Autodesk Fusion 360 part; units mm, degrees
(part 2 of 2)
  arc A410 through (-10.393, 21.7923, -1.2301) (-10.4251, 21.7969, -1.2301) (-10.4574, 21.7984, -1.2301)
  arc A411 through (-24.288, 21.2058, -1.2301) (-24.2358, 20.2463, -1.2301) (-24.1815, 19.2869, -1.2301)
  arc A412 through (-8.9436, 19.8011, -1.2301) (-8.8997, 19.8219, -1.2301) (-8.8672, 19.8581, -1.2301)
  arc A413 through (-23.6188, 17.8727, -1.2301) (-23.6343, 18.3175, -1.2301) (-23.6522, 18.7623, -1.2301)
  arc A414 through (-9.5131, 19.7961, -1.2301) (-9.3106, 19.7881, -1.2301) (-9.108, 19.7825, -1.2301)
  arc A415 through (-8.8381, 19.9649, -1.2301) (-8.8465, 20.0211, -1.2301) (-8.8708, 20.0725, -1.2301)
  arc A416 through (-10.2305, 21.4094, -1.2301) (-10.2433, 21.5149, -1.2301) (-10.2648, 21.619, -1.2301)
  arc A417 through (-8.8672, 19.8581, -1.2301) (-8.8455, 19.9096, -1.2301) (-8.8381, 19.9649, -1.2301)
  arc A418 through (-23.0477, 20.5417, -1.2301) (-22.9869, 20.5553, -1.2301) (-22.9246, 20.5568, -1.2301)
  arc A419 through (-23.9426, 17.1473, -1.2301) (-23.9119, 17.1378, -1.2301) (-23.8802, 17.1321, -1.2301)
  arc A420 through (-24.1815, 19.2869, -1.2301) (-24.1249, 18.3218, -1.2301) (-24.0665, 17.3569, -1.2301)
  arc A421 through (-20.1417, 17.4613, -1.2301) (-20.1217, 17.6929, -1.2301) (-20.123, 17.9253, -1.2301)
  arc A422 through (-29.5876, 20.7478, -1.2301) (-29.7687, 20.7693, -1.2301) (-29.9508, 20.7783, -1.2301)
  arc A423 through (-8.8708, 20.0725, -1.2301) (-8.9093, 20.1152, -1.2301) (-8.9583, 20.1453, -1.2301)
  arc A424 through (-22.2279, 17.2548, -1.2301) (-22.2157, 17.2128, -1.2301) (-22.1903, 17.1771, -1.2301)
  arc A425 through (-22.6634, 20.417, -1.2301) (-22.5849, 20.342, -1.2301) (-22.5222, 20.2535, -1.2301)
  arc A426 through (-22.4438, 20.0412, -1.2301) (-22.4151, 19.8563, -1.2301) (-22.3982, 19.6701, -1.2301)
  line L57 (-10.18, 20.3454, -1.2301) -> (-10.209, 21.0541, -1.2301)
  arc A427 through (-23.2603, 20.4621, -1.2301) (-23.1547, 20.5039, -1.2301) (-23.0477, 20.5417, -1.2301)
  arc A428 through (-23.6237, 17.4644, -1.2301) (-23.6167, 17.6685, -1.2301) (-23.6188, 17.8727, -1.2301)
  arc A429 through (-23.5247, 20.3582, -1.2301) (-23.4617, 20.3815, -1.2301) (-23.3991, 20.4057, -1.2301)
  arc A430 through (-23.987, 17.1766, -1.2301) (-23.9664, 17.1596, -1.2301) (-23.9426, 17.1473, -1.2301)
  arc A431 through (-8.9583, 20.1453, -1.2301) (-9.046, 20.1772, -1.2301) (-9.137, 20.1984, -1.2301)
  arc A432 through (-23.3991, 20.4057, -1.2301) (-23.3295, 20.4336, -1.2301) (-23.2603, 20.4621, -1.2301)
  arc A433 through (-24.0665, 17.3569, -1.2301) (-24.0429, 17.2597, -1.2301) (-23.987, 17.1766, -1.2301)
  arc A434 through (-10.58, 21.7765, -1.2301) (-10.6003, 21.7661, -1.2301) (-10.618, 21.7517, -1.2301)
  arc A435 through (-10.1824, 19.8082, -1.2301) (-10.0878, 19.8088, -1.2301) (-9.9932, 19.809, -1.2301)
  arc A436 through (-21.5279, 20.4378, -1.2301) (-21.3194, 20.4978, -1.2301) (-21.1031, 20.5148, -1.2301)
  arc A437 through (-24.232, 21.4248, -1.2301) (-24.2767, 21.3196, -1.2301) (-24.288, 21.2058, -1.2301)
  arc A438 through (-22.5222, 20.2535, -1.2301) (-22.4741, 20.1506, -1.2301) (-22.4438, 20.0412, -1.2301)
  arc A439 through (-23.6307, 20.3208, -1.2301) (-23.5776, 20.3392, -1.2301) (-23.5247, 20.3582, -1.2301)
  arc A440 through (-22.8153, 20.5219, -1.2301) (-22.7378, 20.4718, -1.2301) (-22.6634, 20.417, -1.2301)
  line L58 (-9.509, 20.2552, -1.2301) -> (-10.18, 20.3454, -1.2301)
  arc A441 through (-29.9508, 20.7783, -1.2301) (-30.1091, 20.7741, -1.2301) (-30.2665, 20.7566, -1.2301)
  arc A442 through (-21.8313, 20.8664, -1.2301) (-21.9495, 20.8378, -1.2301) (-22.07, 20.8212, -1.2301)
  arc A443 through (-20.5452, 17.5083, -1.2301) (-20.5219, 17.4117, -1.2301) (-20.4913, 17.3172, -1.2301)
  arc A444 through (-20.3931, 20.5982, -1.2301) (-20.4399, 20.6955, -1.2301) (-20.5052, 20.7815, -1.2301)
  arc A445 through (-23.744, 20.8149, -1.2301) (-23.7527, 20.818, -1.2301) (-23.7576, 20.8258, -1.2301)
  arc A446 through (-20.3188, 20.319, -1.2301) (-20.35, 20.4602, -1.2301) (-20.3931, 20.5982, -1.2301)
  arc A447 through (-21.2466, 21.0547, -1.2301) (-21.4005, 21.0192, -1.2301) (-21.5495, 20.9666, -1.2301)
  arc A448 through (-20.8881, 10.6636, -1.2301) (-20.8934, 10.6501, -1.2301) (-20.9065, 10.6439, -1.2301)
  arc A449 through (-27.9096, 11.2292, -1.2301) (-27.9142, 11.2191, -1.2301) (-27.9245, 11.2149, -1.2301)
  line L59 (-29.0881, 10.6149, -1.2301) -> (-29.9881, 10.6149, -1.2301)
  arc A450 through (-28.743, 10.6184, -1.2301) (-28.9156, 10.6158, -1.2301) (-29.0881, 10.6149, -1.2301)
  arc A451 through (-23.1426, 13.9894, -1.2301) (-23.1567, 13.9402, -1.2301) (-23.1621, 13.8893, -1.2301)
  arc A452 through (-27.9245, 11.2149, -1.2301) (-27.9375, 11.2179, -1.2301) (-27.948, 11.2262, -1.2301)
  arc A453 through (-28.1881, 10.6636, -1.2301) (-28.1934, 10.6501, -1.2301) (-28.2065, 10.6439, -1.2301)
  line L60 (-29.799, 13.6149, -1.2301) -> (-28.8436, 13.6149, -1.2301)
  arc A454 through (-21.1525, 10.6292, -1.2301) (-21.2977, 10.6226, -1.2301) (-21.443, 10.6184, -1.2301)
  line L61 (-21.7881, 10.6149, -1.2301) -> (-22.6881, 10.6149, -1.2301)
  line L62 (-20.1381, 14.0649, -1.2301) -> (-21.6152, 14.0926, -1.2301)
  arc A455 through (-20.9065, 10.6439, -1.2301) (-21.0295, 10.6362, -1.2301) (-21.1525, 10.6292, -1.2301)
  arc A456 through (-28.7431, 11.4263, -1.2301) (-28.5972, 11.2334, -1.2301) (-28.4525, 11.0398, -1.2301)
  line L63 (-23.1381, 10.1649, -1.2301) -> (-21.6381, 10.1649, -1.2301)
  arc A457 through (-23.1723, 12.7289, -1.2301) (-23.1698, 12.3703, -1.2301) (-23.1655, 12.0117, -1.2301)
  arc A458 through (-22.7937, 14.0871, -1.2301) (-22.9279, 14.0747, -1.2301) (-23.0614, 14.0557, -1.2301)
  line L64 (-21.5799, 12.4149, -1.2301) -> (-22.499, 13.6149, -1.2301)
  line L65 (-28.8799, 12.4149, -1.2301) -> (-29.799, 13.6149, -1.2301)
  line L66 (-20.5881, 13.6149, -1.2301) -> (-20.5881, 12.4149, -1.2301)
  arc A459 through (-27.948, 11.2262, -1.2301) (-28.0841, 11.3968, -1.2301) (-28.2201, 11.5674, -1.2301)
  line L67 (-22.6881, 10.6149, -1.2301) -> (-22.6881, 11.8272, -1.2301)
  arc A460 through (-28.1995, 10.6981, -1.2301) (-28.191, 10.6817, -1.2301) (-28.1881, 10.6636, -1.2301)
  arc A461 through (-20.648, 11.2262, -1.2301) (-20.7841, 11.3968, -1.2301) (-20.9201, 11.5674, -1.2301)
  line L68 (-21.6381, 10.1649, -1.2301) -> (-20.1381, 10.1649, -1.2301)
  arc A462 through (-21.6152, 14.0926, -1.2301) (-21.9888, 14.0982, -1.2301) (-22.3625, 14.1009, -1.2301)
  line L69 (-29.9881, 10.6149, -1.2301) -> (-29.9881, 11.8272, -1.2301)
  arc A463 through (-21.2249, 11.9549, -1.2301) (-21.4028, 12.1846, -1.2301) (-21.5799, 12.4149, -1.2301)
  arc A464 through (-28.2201, 11.5674, -1.2301) (-28.3731, 11.7607, -1.2301) (-28.5249, 11.9549, -1.2301)
  line L70 (-22.499, 13.6149, -1.2301) -> (-21.5436, 13.6149, -1.2301)
  line L71 (-29.9881, 13.0395, -1.2301) -> (-29.0881, 11.8758, -1.2301)
  line L72 (-23.1655, 12.0117, -1.2301) -> (-23.1381, 10.1649, -1.2301)
  arc A465 through (-21.4431, 11.4263, -1.2301) (-21.2972, 11.2334, -1.2301) (-21.1525, 11.0398, -1.2301)
  arc A466 through (-27.8881, 12.4149, -1.2301) (-27.8888, 12.1849, -1.2301) (-27.8907, 11.9548, -1.2301)
  arc A467 through (-21.1525, 11.0398, -1.2301) (-21.0259, 10.869, -1.2301) (-20.8995, 10.6981, -1.2301)
  arc A468 through (-18.1458, 13.994, -1.2301) (-18.1575, 13.8838, -1.2301) (-18.1675, 13.7735, -1.2301)
  arc A469 through (-18.1675, 13.7735, -1.2301) (-18.1769, 13.6401, -1.2301) (-18.183, 13.5064, -1.2301)
  arc A470 through (-18.118, 14.0517, -1.2301) (-18.1368, 14.0252, -1.2301) (-18.1458, 13.994, -1.2301)
  line L73 (-29.9881, 11.8272, -1.2301) -> (-29.9881, 13.0395, -1.2301)
  line L74 (-28.8436, 13.6149, -1.2301) -> (-27.8881, 13.6149, -1.2301)
  line L75 (-22.6881, 13.0395, -1.2301) -> (-21.7881, 11.8758, -1.2301)
  arc A471 through (-27.8907, 11.9548, -1.2301) (-27.8939, 11.7611, -1.2301) (-27.8988, 11.5674, -1.2301)
  arc A472 through (-20.5988, 11.5674, -1.2301) (-20.6041, 11.3983, -1.2301) (-20.6096, 11.2292, -1.2301)
  arc A473 through (-30.3614, 14.0557, -1.2301) (-30.4108, 14.0334, -1.2301) (-30.4426, 13.9894, -1.2301)
  arc A474 through (-28.4525, 11.0398, -1.2301) (-28.3259, 10.869, -1.2301) (-28.1995, 10.6981, -1.2301)
  arc A475 through (-27.8988, 11.5674, -1.2301) (-27.9041, 11.3983, -1.2301) (-27.9096, 11.2292, -1.2301)
  arc A476 through (-28.2065, 10.6439, -1.2301) (-28.3295, 10.6362, -1.2301) (-28.4525, 10.6292, -1.2301)
  arc A477 through (-21.7881, 11.8758, -1.2301) (-21.6152, 11.6514, -1.2301) (-21.4431, 11.4263, -1.2301)
  arc A478 through (-20.9201, 11.5674, -1.2301) (-21.0731, 11.7607, -1.2301) (-21.2249, 11.9549, -1.2301)
  arc A479 through (-20.8995, 10.6981, -1.2301) (-20.891, 10.6817, -1.2301) (-20.8881, 10.6636, -1.2301)
  arc A480 through (-29.0881, 11.8758, -1.2301) (-28.9152, 11.6514, -1.2301) (-28.7431, 11.4263, -1.2301)
  arc A481 through (-20.5907, 11.9548, -1.2301) (-20.5939, 11.7611, -1.2301) (-20.5988, 11.5674, -1.2301)
  arc A482 through (-28.4525, 10.6292, -1.2301) (-28.5977, 10.6226, -1.2301) (-28.743, 10.6184, -1.2301)
  arc A483 through (-20.5881, 12.4149, -1.2301) (-20.5888, 12.1849, -1.2301) (-20.5907, 11.9548, -1.2301)
  arc A484 through (-20.6245, 11.2149, -1.2301) (-20.6375, 11.2179, -1.2301) (-20.648, 11.2262, -1.2301)
  arc A485 through (-23.17, 13.3545, -1.2301) (-23.1724, 13.0417, -1.2301) (-23.1723, 12.7289, -1.2301)
  arc A486 through (-21.443, 10.6184, -1.2301) (-21.6156, 10.6158, -1.2301) (-21.7881, 10.6149, -1.2301)
  line L76 (-20.1381, 10.1649, -1.2301) -> (-20.1381, 12.1149, -1.2301)
  line L77 (-22.6881, 11.8272, -1.2301) -> (-22.6881, 13.0395, -1.2301)
  arc A487 through (-22.3625, 14.1009, -1.2301) (-22.5782, 14.0978, -1.2301) (-22.7937, 14.0871, -1.2301)
  arc A488 through (-23.0614, 14.0557, -1.2301) (-23.1108, 14.0334, -1.2301) (-23.1426, 13.9894, -1.2301)
  arc A489 through (-28.5249, 11.9549, -1.2301) (-28.7028, 12.1846, -1.2301) (-28.8799, 12.4149, -1.2301)
  arc A490 through (-20.6096, 11.2292, -1.2301) (-20.6142, 11.2191, -1.2301) (-20.6245, 11.2149, -1.2301)
  arc A491 through (-23.1621, 13.8893, -1.2301) (-23.1665, 13.6219, -1.2301) (-23.17, 13.3545, -1.2301)
  line L78 (-27.8881, 13.6149, -1.2301) -> (-27.8881, 12.4149, -1.2301)
  arc A492 through (-30.0937, 14.0871, -1.2301) (-30.2279, 14.0747, -1.2301) (-30.3614, 14.0557, -1.2301)
  line L79 (-20.1381, 12.1149, -1.2301) -> (-20.1381, 14.0649, -1.2301)
  line L80 (-21.5436, 13.6149, -1.2301) -> (-20.5881, 13.6149, -1.2301)
  arc A493 through (-18.0469, 10.2033, -1.2301) (-17.9958, 10.1748, -1.2301) (-17.9381, 10.1649, -1.2301)
  arc A494 through (-16.7055, 12.3715, -1.2301) (-16.8822, 12.3846, -1.2301) (-17.0592, 12.3946, -1.2301)
  line L81 (-18.1958, 11.9056, -1.2301) -> (-18.1669, 11.0353, -1.2301)
  line L82 (-18.8169, 11.9353, -1.2301) -> (-18.1958, 11.9056, -1.2301)
  line L83 (-17.6805, 11.9056, -1.2301) -> (-17.0593, 11.9353, -1.2301)
  line L84 (-18.1881, 13.203, -1.2301) -> (-18.1881, 12.4245, -1.2301)
  arc A495 through (-18.183, 13.5064, -1.2301) (-18.1868, 13.3548, -1.2301) (-18.1881, 13.203, -1.2301)
  arc A496 through (-19.3313, 12.3358, -1.2301) (-19.3756, 12.3102, -1.2301) (-19.4089, 12.2713, -1.2301)
  arc A497 through (-16.5445, 11.9941, -1.2301) (-16.5003, 12.0197, -1.2301) (-16.4672, 12.0586, -1.2301)
  arc A498 through (-19.1707, 11.9584, -1.2301) (-18.9939, 11.9453, -1.2301) (-18.8169, 11.9353, -1.2301)
  arc A499 through (-19.4091, 12.0586, -1.2301) (-19.376, 12.0197, -1.2301) (-19.3318, 11.9941, -1.2301)
  arc A500 through (-10.3041, 13.1503, -1.2301) (-10.1609, 13.1636, -1.2301) (-10.0192, 13.1876, -1.2301)
  arc A501 through (-16.5445, 12.3358, -1.2301) (-16.6237, 12.3591, -1.2301) (-16.7055, 12.3715, -1.2301)
  arc A502 through (-17.0593, 11.9353, -1.2301) (-16.8823, 11.9453, -1.2301) (-16.7055, 11.9584, -1.2301)
  arc A503 through (-15.1512, 10.2264, -1.2301) (-15.1025, 10.1813, -1.2301) (-15.0381, 10.1649, -1.2301)
  arc A504 through (-16.7055, 11.9584, -1.2301) (-16.6238, 11.9707, -1.2301) (-16.5445, 11.9941, -1.2301)
  arc A505 through (-18.023, 14.0926, -1.2301) (-18.0519, 14.0859, -1.2301) (-18.08, 14.0765, -1.2301)
  arc A506 through (-10.4908, 10.2591, -1.2301) (-10.2893, 10.2689, -1.2301) (-10.0887, 10.2893, -1.2301)
  line L85 (-17.7093, 11.0353, -1.2301) -> (-17.6805, 11.9056, -1.2301)
  arc A507 through (-17.7317, 10.5158, -1.2301) (-17.7192, 10.7755, -1.2301) (-17.7093, 11.0353, -1.2301)
  arc A508 through (-16.4672, 12.0586, -1.2301) (-16.4455, 12.1098, -1.2301) (-16.4381, 12.1649, -1.2301)
  arc A509 through (-12.7902, 11.1668, -1.2301) (-12.7379, 11.3526, -1.2301) (-12.6848, 11.5381, -1.2301)
  arc A510 through (-17.7305, 13.6633, -1.2301) (-17.7428, 13.7827, -1.2301) (-17.7639, 13.901, -1.2301)
  arc A511 through (-18.1111, 10.3023, -1.2301) (-18.0869, 10.2476, -1.2301) (-18.0469, 10.2033, -1.2301)
  arc A512 through (-10.407, 10.6709, -1.2301) (-10.885, 10.6828, -1.2301) (-11.3631, 10.6925, -1.2301)
  arc A513 through (-19.4381, 12.1649, -1.2301) (-19.4307, 12.1098, -1.2301) (-19.4091, 12.0586, -1.2301)
  arc A514 through (-12.8596, 10.7627, -1.2301) (-12.8791, 10.7722, -1.2301) (-12.8867, 10.7925, -1.2301)
  arc A515 through (-19.1694, 12.3715, -1.2301) (-19.2516, 12.3592, -1.2301) (-19.3313, 12.3358, -1.2301)
  arc A516 through (-15.0134, 13.5959, -1.2301) (-15.0488, 13.6, -1.2301) (-15.0843, 13.5986, -1.2301)
  arc A517 through (-16.4672, 12.2712, -1.2301) (-16.5003, 12.3102, -1.2301) (-16.5445, 12.3358, -1.2301)
  line L86 (-18.1881, 12.4245, -1.2301) -> (-18.8131, 12.3947, -1.2301)
  arc A518 through (-17.9381, 10.1649, -1.2301) (-17.8805, 10.1748, -1.2301) (-17.8294, 10.2033, -1.2301)
  arc A519 through (-17.7651, 10.3023, -1.2301) (-17.743, 10.4082, -1.2301) (-17.7317, 10.5158, -1.2301)
  arc A520 through (-18.8131, 12.3947, -1.2301) (-18.9914, 12.3847, -1.2301) (-19.1694, 12.3715, -1.2301)
  arc A521 through (-18.1669, 11.0353, -1.2301) (-18.157, 10.7755, -1.2301) (-18.1445, 10.5158, -1.2301)
  arc A522 through (-18.1445, 10.5158, -1.2301) (-18.1332, 10.4082, -1.2301) (-18.1111, 10.3023, -1.2301)
  arc A523 through (-9.8894, 13.4761, -1.2301) (-9.9521, 13.5166, -1.2301) (-10.0231, 13.5395, -1.2301)
  arc A524 through (-15.0381, 10.1649, -1.2301) (-14.9733, 10.182, -1.2301) (-14.9253, 10.2288, -1.2301)
  arc A525 through (-10.0231, 13.5395, -1.2301) (-10.169, 13.5606, -1.2301) (-10.3161, 13.571, -1.2301)
  arc A526 through (-13.0848, 11.9529, -1.2301) (-13.2769, 11.3044, -1.2301) (-13.4636, 10.6545, -1.2301)
  arc A527 through (-15.2726, 12.3824, -1.2301) (-15.2702, 12.0716, -1.2301) (-15.2658, 11.7609, -1.2301)
  arc A528 through (-19.3318, 11.9941, -1.2301) (-19.2525, 11.9707, -1.2301) (-19.1707, 11.9584, -1.2301)
  arc A529 through (-12.5967, 10.2277, -1.2301) (-12.106, 10.2314, -1.2301) (-11.6154, 10.2376, -1.2301)
  arc A530 through (-16.4381, 12.1649, -1.2301) (-16.4455, 12.22, -1.2301) (-16.4672, 12.2712, -1.2301)
  arc A531 through (-17.893, 14.0923, -1.2301) (-17.9251, 14.0969, -1.2301) (-17.9574, 14.0984, -1.2301)
  arc A532 through (-19.4089, 12.2713, -1.2301) (-19.4307, 12.2201, -1.2301) (-19.4381, 12.1649, -1.2301)
  arc A533 through (-9.8882, 13.2535, -1.2301) (-9.8512, 13.3039, -1.2301) (-9.8381, 13.3649, -1.2301)
  arc A534 through (-12.879, 10.8461, -1.2301) (-12.8347, 11.0065, -1.2301) (-12.7902, 11.1668, -1.2301)
  arc A535 through (-17.8294, 10.2033, -1.2301) (-17.7893, 10.2476, -1.2301) (-17.7651, 10.3023, -1.2301)
  line L87 (-12.2347, 13.0649, -1.2301) -> (-11.0364, 13.1149, -1.2301)
  arc A536 through (-13.0794, 10.2426, -1.2301) (-12.8382, 10.2308, -1.2301) (-12.5967, 10.2277, -1.2301)
  arc A537 through (-14.8662, 13.2955, -1.2301) (-14.8843, 13.4057, -1.2301) (-14.9158, 13.5127, -1.2301)
  arc A538 through (-15.1526, 13.5797, -1.2301) (-15.1817, 13.5636, -1.2301) (-15.2078, 13.5428, -1.2301)
  arc A539 through (-12.4397, 10.7333, -1.2301) (-12.6497, 10.7475, -1.2301) (-12.8596, 10.7627, -1.2301)
  arc A540 through (-12.5086, 13.4927, -1.2301) (-12.6164, 13.3803, -1.2301) (-12.6856, 13.2408, -1.2301)
  arc A541 through (-11.0364, 13.1149, -1.2301) (-10.6702, 13.1314, -1.2301) (-10.3041, 13.1503, -1.2301)
  arc A542 through (-17.9574, 14.0984, -1.2301) (-17.9903, 14.0969, -1.2301) (-18.023, 14.0926, -1.2301)
  arc A543 through (-9.8381, 10.4649, -1.2301) (-9.8539, 10.5287, -1.2301) (-9.8976, 10.5776, -1.2301)
  arc A544 through (-15.2658, 11.7609, -1.2301) (-15.256, 11.2591, -1.2301) (-15.2441, 10.7574, -1.2301)
  arc A545 through (-9.8381, 13.3649, -1.2301) (-9.8516, 13.4261, -1.2301) (-9.8894, 13.4761, -1.2301)
  arc A546 through (-13.4636, 10.6545, -1.2301) (-13.4808, 10.5065, -1.2301) (-13.4503, 10.3606, -1.2301)
  arc A547 through (-9.9044, 10.3508, -1.2301) (-9.8559, 10.3989, -1.2301) (-9.8381, 10.4649, -1.2301)
  arc A548 through (-14.8381, 11.8636, -1.2301) (-14.8393, 12.3675, -1.2301) (-14.8428, 12.8714, -1.2301)
  arc A549 through (-11.6154, 10.2376, -1.2301) (-11.0531, 10.2473, -1.2301) (-10.4908, 10.2591, -1.2301)
  arc A550 through (-10.0887, 10.2893, -1.2301) (-9.9935, 10.311, -1.2301) (-9.9044, 10.3508, -1.2301)
  line L88 (-17.0592, 12.3946, -1.2301) -> (-17.6802, 12.4243, -1.2301)
  arc A551 through (-15.0843, 13.5986, -1.2301) (-15.1192, 13.5918, -1.2301) (-15.1526, 13.5797, -1.2301)
  arc A552 through (-10.0192, 13.1876, -1.2301) (-9.9493, 13.212, -1.2301) (-9.8882, 13.2535, -1.2301)
  arc A553 through (-15.2699, 12.9281, -1.2301) (-15.2725, 12.6553, -1.2301) (-15.2726, 12.3824, -1.2301)
  arc A554 through (-18.08, 14.0765, -1.2301) (-18.1003, 14.0661, -1.2301) (-18.118, 14.0517, -1.2301)
  arc A555 through (-15.2411, 13.4933, -1.2301) (-15.2555, 13.4431, -1.2301) (-15.2612, 13.3913, -1.2301)
  arc A556 through (-14.8428, 12.8714, -1.2301) (-14.8497, 13.0838, -1.2301) (-14.8662, 13.2955, -1.2301)
  arc A557 through (-11.3631, 10.6925, -1.2301) (-11.6555, 10.6991, -1.2301) (-11.9478, 10.7083, -1.2301)
  arc A558 through (-15.2078, 13.5428, -1.2301) (-15.2272, 13.5199, -1.2301) (-15.2411, 13.4933, -1.2301)
  arc A559 through (-14.9253, 10.2288, -1.2301) (-14.8865, 10.3124, -1.2301) (-14.8661, 10.4023, -1.2301)
  line L89 (-17.6802, 12.4243, -1.2301) -> (-17.7092, 13.2435, -1.2301)
  arc A560 through (-10.3161, 13.571, -1.2301) (-10.7031, 13.583, -1.2301) (-11.0902, 13.5927, -1.2301)
  arc A561 through (-12.6856, 13.2408, -1.2301) (-12.8879, 12.5977, -1.2301) (-13.0848, 11.9529, -1.2301)
  arc A562 through (-13.3545, 10.2796, -1.2301) (-13.2176, 10.2565, -1.2301) (-13.0794, 10.2426, -1.2301)
  arc A563 through (-15.2612, 13.3913, -1.2301) (-15.2661, 13.1597, -1.2301) (-15.2699, 12.9281, -1.2301)
  arc A564 through (-9.8976, 10.5776, -1.2301) (-9.9739, 10.6179, -1.2301) (-10.0572, 10.6402, -1.2301)
  arc A565 through (-12.8867, 10.7925, -1.2301) (-12.8845, 10.8195, -1.2301) (-12.879, 10.8461, -1.2301)
  arc A566 through (-15.2135, 10.3929, -1.2301) (-15.1914, 10.3063, -1.2301) (-15.1512, 10.2264, -1.2301)
  arc A567 through (-17.8149, 14.036, -1.2301) (-17.8477, 14.0728, -1.2301) (-17.893, 14.0923, -1.2301)
  arc A568 through (-15.2441, 10.7574, -1.2301) (-15.2341, 10.5747, -1.2301) (-15.2135, 10.3929, -1.2301)
  arc A569 through (-10.0572, 10.6402, -1.2301) (-10.2316, 10.6608, -1.2301) (-10.407, 10.6709, -1.2301)
  arc A570 through (-14.8661, 10.4023, -1.2301) (-14.8489, 10.5928, -1.2301) (-14.8422, 10.7841, -1.2301)
  arc A571 through (-13.4503, 10.3606, -1.2301) (-13.4128, 10.3078, -1.2301) (-13.3545, 10.2796, -1.2301)
  line L90 (-12.56, 11.9649, -1.2301) -> (-12.2347, 13.0649, -1.2301)
  arc A572 through (-11.9478, 10.7083, -1.2301) (-12.1938, 10.719, -1.2301) (-12.4397, 10.7333, -1.2301)
  arc A573 through (-17.7092, 13.2435, -1.2301) (-17.7182, 13.4535, -1.2301) (-17.7305, 13.6633, -1.2301)
  arc A574 through (-14.8422, 10.7841, -1.2301) (-14.8391, 11.3238, -1.2301) (-14.8381, 11.8636, -1.2301)
  arc A575 through (-12.6848, 11.5381, -1.2301) (-12.6227, 11.7516, -1.2301) (-12.56, 11.9649, -1.2301)
  arc A576 through (-14.9158, 13.5127, -1.2301) (-14.9537, 13.5672, -1.2301) (-15.0134, 13.5959, -1.2301)
  arc A577 through (-17.7639, 13.901, -1.2301) (-17.7844, 13.9703, -1.2301) (-17.8149, 14.036, -1.2301)
  arc A578 through (-12.3707, 13.5523, -1.2301) (-12.4434, 13.5311, -1.2301) (-12.5086, 13.4927, -1.2301)
  arc A579 through (-5.303, 17.8735, -1.2301) (-5.3191, 18.4384, -1.2301) (-5.3405, 19.0032, -1.2301)
  arc A580 through (-5.439, 17.1788, -1.2301) (-5.3695, 17.2704, -1.2301) (-5.3339, 17.3797, -1.2301)
  arc A581 through (-7.9514, 16.9186, -1.2301) (-7.8874, 16.9218, -1.2301) (-7.8258, 16.9395, -1.2301)
  arc A582 through (-6.9071, 20.8063, -1.2301) (-6.7489, 20.8111, -1.2301) (-6.5938, 20.7795, -1.2301)
  arc A583 through (-12.0919, 13.5847, -1.2301) (-12.2317, 13.5716, -1.2301) (-12.3707, 13.5523, -1.2301)
  arc A584 through (-5.7471, 17.5199, -1.2301) (-5.7247, 17.3753, -1.2301) (-5.6952, 17.232, -1.2301)
  line L91 (-5.9074, 20.4105, -1.2301) -> (-5.8346, 18.8045, -1.2301)
  line L92 (-5.3405, 19.0032, -1.2301) -> (-5.4135, 20.7108, -1.2301)
  arc A585 through (-7.5304, 20.4229, -1.2301) (-7.3761, 20.5652, -1.2301) (-7.2079, 20.6906, -1.2301)
  line L93 (-5.4135, 20.7108, -1.2301) -> (-5.8722, 20.9796, -1.2301)
  arc A586 through (-7.7388, 17.0138, -1.2301) (-7.7224, 17.0517, -1.2301) (-7.7174, 17.0928, -1.2301)
  arc A587 through (-5.8722, 20.9796, -1.2301) (-5.9752, 21.0359, -1.2301) (-6.0815, 21.0858, -1.2301)
  arc A588 through (-5.8346, 18.8045, -1.2301) (-5.8145, 18.3956, -1.2301) (-5.7915, 17.9868, -1.2301)
  arc A589 through (-5.6182, 17.1435, -1.2301) (-5.5235, 17.1353, -1.2301) (-5.439, 17.1788, -1.2301)
  arc A590 through (-11.6862, 13.5991, -1.2301) (-11.8892, 13.5954, -1.2301) (-12.0919, 13.5847, -1.2301)
  arc A591 through (-8.4899, 21.1855, -1.2301) (-8.3522, 19.2872, -1.2301) (-8.2134, 17.389, -1.2301)
  arc A592 through (-7.2079, 20.6906, -1.2301) (-7.0639, 20.7652, -1.2301) (-6.9071, 20.8063, -1.2301)
  line L94 (-6.2345, 20.6127, -1.2301) -> (-5.9074, 20.4105, -1.2301)
  arc A593 through (-5.6952, 17.232, -1.2301) (-5.6678, 17.1781, -1.2301) (-5.6182, 17.1435, -1.2301)
  arc A594 through (-5.3339, 17.3797, -1.2301) (-5.3078, 17.6259, -1.2301) (-5.303, 17.8735, -1.2301)
  arc A595 through (-8.7308, 25.2268, -1.2301) (-8.7625, 25.1512, -1.2301) (-8.7695, 25.0694, -1.2301)
  arc A596 through (-11.0902, 13.5927, -1.2301) (-11.3882, 13.5976, -1.2301) (-11.6862, 13.5991, -1.2301)
  line L95 (-7.9132, 20.0308, -1.2301) -> (-7.5304, 20.4229, -1.2301)
  arc A597 through (-8.7695, 25.0694, -1.2301) (-8.63, 23.1274, -1.2301) (-8.4899, 21.1855, -1.2301)
  arc A598 through (-7.7547, 18.0055, -1.2301) (-7.7738, 18.2887, -1.2301) (-7.7954, 18.5718, -1.2301)
  arc A599 through (-33.8381, 22.9018, -1.2301) (-34.111, 22.8838, -1.2301) (-34.3838, 22.8645, -1.2301)
  arc A600 through (-27.0705, 23.1748, -1.2301) (-26.9835, 22.0437, -1.2301) (-26.8957, 20.9126, -1.2301)
  arc A601 through (-26.8957, 20.9126, -1.2301) (-26.8143, 19.895, -1.2301) (-26.7287, 18.8776, -1.2301)
  arc A602 through (-35.4029, 20.2744, -1.2301) (-35.3569, 19.4444, -1.2301) (-35.3035, 18.6149, -1.2301)
  arc A603 through (-35.4542, 22.6398, -1.2301) (-35.4522, 22.1115, -1.2301) (-35.4462, 21.5832, -1.2301)
  arc A604 through (-25.7292, 17.7001, -1.2301) (-25.8567, 17.7153, -1.2301) (-25.9629, 17.7874, -1.2301)
  arc A605 through (-7.7302, 17.5123, -1.2301) (-7.7408, 17.7589, -1.2301) (-7.7547, 18.0055, -1.2301)
  arc A606 through (-25.082, 17.7409, -1.2301) (-25.1883, 17.7492, -1.2301) (-25.2949, 17.7457, -1.2301)
  arc A607 through (-8.1393, 17.0399, -1.2301) (-8.112, 16.9918, -1.2301) (-8.0702, 16.9557, -1.2301)
  arc A608 through (-35.1482, 17.707, -1.2301) (-35.0971, 17.6758, -1.2301) (-35.0381, 17.6649, -1.2301)
  arc A609 through (-7.8258, 16.9395, -1.2301) (-7.7765, 16.9699, -1.2301) (-7.7388, 17.0138, -1.2301)
  arc A610 through (-5.7915, 17.9868, -1.2301) (-5.7734, 17.7529, -1.2301) (-5.7471, 17.5199, -1.2301)
  arc A611 through (-6.3319, 21.1825, -1.2301) (-6.4568, 21.2221, -1.2301) (-6.5831, 21.2566, -1.2301)
  line L96 (-7.7954, 18.5718, -1.2301) -> (-7.9132, 20.0308, -1.2301)
  arc A612 through (-35.3662, 22.7661, -1.2301) (-35.43, 22.7168, -1.2301) (-35.4542, 22.6398, -1.2301)
  arc A613 through (-8.5717, 25.2989, -1.2301) (-8.6056, 25.2952, -1.2301) (-8.6388, 25.2875, -1.2301)
  arc A614 through (-8.0702, 16.9557, -1.2301) (-8.013, 16.93, -1.2301) (-7.9514, 16.9186, -1.2301)
  line L97 (-7.9613, 20.7178, -1.2301) -> (-8.0894, 22.4914, -1.2301)
  arc A615 through (-24.9086, 17.5902, -1.2301) (-24.9298, 17.6455, -1.2301) (-24.9681, 17.6906, -1.2301)
  arc A616 through (-35.3035, 18.6149, -1.2301) (-35.2828, 18.3333, -1.2301) (-35.2594, 18.0519, -1.2301)
  arc A617 through (-26.7287, 18.8776, -1.2301) (-26.6814, 18.4225, -1.2301) (-26.6182, 17.9693, -1.2301)
  arc A618 through (-6.7933, 21.2928, -1.2301) (-6.9268, 21.3023, -1.2301) (-7.0607, 21.3053, -1.2301)
  arc A619 through (-35.0381, 17.6649, -1.2301) (-34.9773, 17.6786, -1.2301) (-34.9282, 17.7171, -1.2301)
  arc A620 through (-26.5768, 17.8001, -1.2301) (-26.5431, 17.7087, -1.2301) (-26.504, 17.6195, -1.2301)
  arc A621 through (-34.9282, 17.7171, -1.2301) (-34.8901, 17.7799, -1.2301) (-34.8708, 17.8508, -1.2301)
  arc A622 through (-26.1765, 17.2132, -1.2301) (-26.1185, 17.1776, -1.2301) (-26.0551, 17.1529, -1.2301)
  arc A623 through (-8.3739, 25.1788, -1.2301) (-8.423, 25.2543, -1.2301) (-8.5038, 25.2941, -1.2301)
  arc A624 through (-8.214, 24.1411, -1.2301) (-8.2468, 24.4826, -1.2301) (-8.2913, 24.8228, -1.2301)
  arc A625 through (-6.0815, 21.0858, -1.2301) (-6.2057, 21.1367, -1.2301) (-6.3319, 21.1825, -1.2301)
  arc A626 through (-6.5938, 20.7795, -1.2301) (-6.4092, 20.7068, -1.2301) (-6.2345, 20.6127, -1.2301)
  arc A627 through (-6.5831, 21.2566, -1.2301) (-6.6875, 21.2786, -1.2301) (-6.7933, 21.2928, -1.2301)
  arc A628 through (-35.2166, 17.8168, -1.2301) (-35.1903, 17.757, -1.2301) (-35.1482, 17.707, -1.2301)
  arc A629 through (-34.8708, 17.8508, -1.2301) (-34.8572, 17.9996, -1.2301) (-34.8541, 18.1491, -1.2301)
  arc A630 through (-7.7174, 17.0928, -1.2301) (-7.7232, 17.3025, -1.2301) (-7.7302, 17.5123, -1.2301)
  arc A631 through (-26.7234, 23.3927, -1.2301) (-26.7811, 23.408, -1.2301) (-26.8406, 23.412, -1.2301)
  arc A632 through (-34.8541, 18.1491, -1.2301) (-34.8612, 18.5666, -1.2301) (-34.8704, 18.984, -1.2301)
  arc A633 through (-35.2594, 18.0519, -1.2301) (-35.2434, 17.9334, -1.2301) (-35.2166, 17.8168, -1.2301)
  arc A634 through (-26.2077, 18.7305, -1.2301) (-26.2985, 19.7429, -1.2301) (-26.3857, 20.7556, -1.2301)
  arc A635 through (-8.2134, 17.389, -1.2301) (-8.1882, 17.2119, -1.2301) (-8.1393, 17.0399, -1.2301)
  arc A636 through (-7.2371, 21.2771, -1.2301) (-7.3202, 21.2427, -1.2301) (-7.397, 21.1959, -1.2301)
  arc A637 through (-7.0607, 21.3053, -1.2301) (-7.15, 21.2981, -1.2301) (-7.2371, 21.2771, -1.2301)
  arc A638 through (-26.6182, 17.9693, -1.2301) (-26.6011, 17.8838, -1.2301) (-26.5768, 17.8001, -1.2301)
  arc A639 through (-25.2949, 17.7457, -1.2301) (-25.5123, 17.7246, -1.2301) (-25.7292, 17.7001, -1.2301)
  arc A640 through (-8.0894, 22.4914, -1.2301) (-8.1503, 23.3163, -1.2301) (-8.214, 24.1411, -1.2301)
  arc A641 through (-25.7219, 17.1614, -1.2301) (-25.5214, 17.2026, -1.2301) (-25.3224, 17.2508, -1.2301)
  arc A642 through (-26.4129, 17.4546, -1.2301) (-26.368, 17.3917, -1.2301) (-26.3165, 17.3342, -1.2301)
  arc A643 through (-26.0551, 17.1529, -1.2301) (-25.9867, 17.1392, -1.2301) (-25.917, 17.1374, -1.2301)
  arc A644 through (-24.939, 17.4599, -1.2301) (-24.9097, 17.5217, -1.2301) (-24.9086, 17.5902, -1.2301)
  arc A645 through (-26.504, 17.6195, -1.2301) (-26.461, 17.5356, -1.2301) (-26.4129, 17.4546, -1.2301)
  arc A646 through (-25.3224, 17.2508, -1.2301) (-25.1941, 17.2923, -1.2301) (-25.0713, 17.3483, -1.2301)
  arc A647 through (-26.47, 21.7165, -1.2301) (-26.5086, 22.1281, -1.2301) (-26.5493, 22.5394, -1.2301)
  arc A648 through (-26.6235, 23.2594, -1.2301) (-26.6317, 23.2964, -1.2301) (-26.6478, 23.3306, -1.2301)
  arc A649 through (-24.9681, 17.6906, -1.2301) (-25.0215, 17.7239, -1.2301) (-25.082, 17.7409, -1.2301)
  line L98 (-34.8704, 18.984, -1.2301) -> (-34.9027, 20.3031, -1.2301)
  arc A650 through (-26.6478, 23.3306, -1.2301) (-26.6805, 23.3679, -1.2301) (-26.7234, 23.3927, -1.2301)
  arc A651 through (-34.8645, 22.8254, -1.2301) (-35.0681, 22.8069, -1.2301) (-35.2716, 22.7877, -1.2301)
  arc A652 through (-35.4462, 21.5832, -1.2301) (-35.4304, 20.9286, -1.2301) (-35.4029, 20.2744, -1.2301)
  arc A653 through (-7.397, 21.1959, -1.2301) (-7.5048, 21.1143, -1.2301) (-7.6085, 21.0275, -1.2301)
  arc A654 through (-25.9629, 17.7874, -1.2301) (-26.0532, 17.918, -1.2301) (-26.1066, 18.0675, -1.2301)
  arc A655 through (-8.5038, 25.2941, -1.2301) (-8.5376, 25.2986, -1.2301) (-8.5717, 25.2989, -1.2301)
  line L99 (-7.6085, 21.0275, -1.2301) -> (-7.9613, 20.7178, -1.2301)
  arc A656 through (-25.917, 17.1374, -1.2301) (-25.8191, 17.1463, -1.2301) (-25.7219, 17.1614, -1.2301)
  arc A657 through (-8.6388, 25.2875, -1.2301) (-8.6678, 25.2768, -1.2301) (-8.6951, 25.2624, -1.2301)
  arc A658 through (-25.0713, 17.3483, -1.2301) (-24.9991, 17.3969, -1.2301) (-24.939, 17.4599, -1.2301)
  arc A659 through (-8.2913, 24.8228, -1.2301) (-8.3253, 25.0025, -1.2301) (-8.3739, 25.1788, -1.2301)
extrude "Extrude5" cut sketch "falmouthrobotics" against normal blind 0.3 contours A0 A1 A4 A5 A6 A7 A11 A12 A14 L4 L5 A15 A16 A17 A18 A20 A22 A24 A25 A27 A30 A31 A35 A37 L12 A39 L13 A45 A51 A52 A53 A55 L16 A56 A57 A58 A59 L17 L18 A60 A61 A62 A63 A64 A65 A66 A67 A69 A70 A71 L22 A72 A73 A75 A76 A242 | A2 L0 L1 A9 L2 A13 L3 L8 A26 L9 A28 A32 A33 L10 A36 L11 A40 A41 A42 A43 A46 A48 L14 A50 A177 A182 A189 A197 A205 A207 L40 A220 A224 A229 A230 A231 A232 A235 A236 A239 A241 A247 | A3 A8 A10 A19 A29 A34 A38 A44 A47 A226 A227 A233 A234 A237 A238 A240 | L6 L7 A21 A23 A49 A54 L15 L19 L20 A68 L21 A74 A473 A492 | A77 A78 A79 A80 A84 A85 A88 A89 A90 A91 A93 A97 A98 A99 A100 A101 A102 A104 A106 A107 A110 A111 A112 A113 A114 A116 A119 A122 A123 A143 A148 A149 A375 A376 A382 A383 L55 A385 A386 A388 A389 A391 A392 A393 A395 A396 A397 A399 A401 A402 L56 A404 A405 A406 A407 A409 A411 A413 A418 A419 A420 A421 A424 A425 A426 A427 A428 A429 A430 A432 A433 A436 A437 A438 A439 A440 A442 A443 A444 A445 A446 A447 | A81 A82 A83 L23 A86 A87 A92 A94 A95 A96 A103 A105 A108 A109 L24 A115 A117 A118 A120 A121 A130 A136 A142 A146 A147 A151 A152 A155 A156 A159 A160 A162 A165 A166 A171 A172 A193 A194 A214 A219 A422 A441 | A125 A126 A128 A131 A140 A141 A145 A153 A154 A158 A164 A167 A169 A173 A191 A215 | A174 A176 A179 A183 L36 A204 L37 L39 A211 A212 L41 A223 L43 A225 L44 L45 L46 A243 A245 A246 | A248 A249 A250 A251 A252 A258 A259 A600 A601 A604 A606 A615 A617 A620 A622 A631 A634 A638 A639 A641 A642 A643 A644 A645 A646 A647 A648 A649 A650 A654 A656 A658 | A253 A579 A580 A581 A582 A584 L91 L92 A585 L93 A586 A587 A588 A589 A591 A592 L94 A593 A594 A595 L95 A597 A598 A605 A607 A609 A610 A611 L96 A613 A614 L97 A618 A623 A624 A625 A626 A627 A630 A635 A636 A637 A640 A653 A655 L99 A657 A659 | A254 A256 A257 A262 A263 A264 L48 A266 A267 A268 A269 A270 A274 A276 A278 A280 A281 A283 A287 A288 L49 A290 A291 A294 A296 A297 A298 A299 A301 A302 A303 A304 A305 A306 A307 A310 A320 A322 A324 L51 A329 A599 A602 A603 A608 A612 A616 A619 A621 A628 A629 A632 A633 L98 A651 A652 | A255 A260 A261 A265 A271 A272 A273 A275 A277 A279 A282 A284 A285 A286 A289 A292 A293 A295 A300 A308 A309 A311 A312 A313 A315 A316 A317 A318 A323 A325 A327 A328 A330 A331 A333 A334 A335 A336 A337 A339 A345 A346 A348 A349 A350 A351 A352 A355 A356 A357 A358 A359 A362 A363 A366 A367 A370 A373 A374 A378 | A314 A319 A321 L50 A326 A332 A338 L52 A340 A341 A342 A343 A344 A347 L53 A353 A354 A360 L54 A361 A364 A365 A368 A369 A371 A372 A377 A379 A380 A381 A384 A387 A390 A394 A398 A400 A403 A408 A410 A412 A414 A415 A416 A417 A423 L57 A431 A434 A435 L58 | A451 L62 L63 A457 A458 L68 A462 L72 A485 L76 A487 A488 A491 L79 | A468 A469 A470 A493 A494 L81 L82 L83 L84 A495 A496 A497 A498 A499 A501 A502 A504 A505 L85 A507 A508 A510 A511 A513 A515 A517 L86 A518 A519 A520 A521 A522 A528 A530 A531 A532 A535 A542 L88 A554 L89 A567 A573 A577 | A500 A506 A509 A512 A514 A523 A525 A526 A529 A533 A534 L87 A536 A539 A540 A541 A543 A545 A546 A547 A549 A550 A552 A557 A560 A561 A562 A564 A565 A569 A571 L90 A572 A575 A578 A583 A590 A596 | A503 A516 A524 A527 A537 A538 A544 A548 A551 A553 A555 A556 A558 A559 A563 A566 A568 A570 A574 A576 in plane through (0, 0, 1.2301) normal (0, 0, -1)
